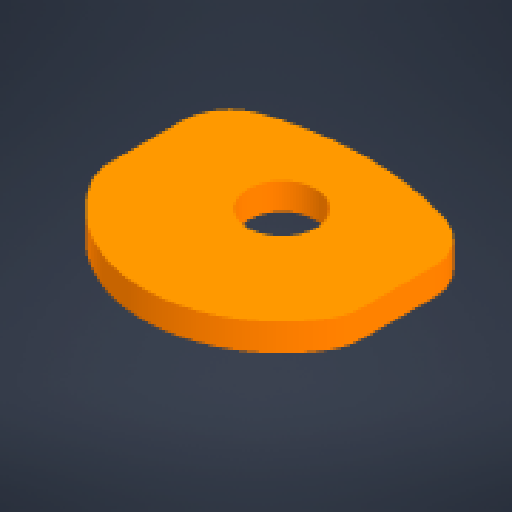
# Autodesk Inventor part: gasket_1
Saved by Autodesk Inventor 2024 (Build 280153000, 153)
## iProperties
Created: 2023-11-08
Part Number: gasket_1
Material: Типовые
Document SubType Name: Modeling
Designer: user
Density: 1 g/cm^3
Appearance: По умолчанию
Author: user
Autodesk Inventor part; units mm, degrees
ref_plane "YZ Plane" through (0, 0, 0) normal (1, 0, 0) x (0, 1, 0)
ref_plane "XZ Plane" through (0, 0, 0) normal (0, 1, 0) x (-1, 0, 0)
ref_plane "XY Plane" through (0, 0, 0) normal (0, 0, 1) x (1, 0, 0)
sketch "Эскиз1" plane through (0, 0, 0) normal (0, 0, 1) x (1, 0, 0)
  circle A0 centre (-3.5, 33.9378) radius 1.5 projected
  circle A1 centre (7, 40) radius 1.5 projected
  circle A2 centre (-7, 40) radius 1.5 projected
  circle A3 centre (3.5, 33.9378) radius 1.5 projected
  arc A4 (9.6, 47.3855) -> (-9.6, 47.3855) centre (0, 18.963) ccw projected
  line L0 (-13, 42.6484) -> (-13, 35.2228) projected
  arc A5 (-12.2928, 32.6593) -> (12.2928, 32.6593) centre (0, 40) ccw projected
  line L1 (13, 35.2228) -> (13, 42.6484) projected
  circle A6 centre (0, 40) radius 3.1 projected
  arc A7 (12.2928, 32.6593) -> (13, 35.2228) centre (8, 35.2228) ccw projected
  arc A8 (13, 42.6484) -> (9.6, 47.3855) centre (8, 42.6484) ccw projected
  arc A9 (-9.6, 47.3855) -> (-13, 42.6484) centre (-8, 42.6484) ccw projected
  arc A10 (-13, 35.2228) -> (-12.2928, 32.6593) centre (-8, 35.2228) ccw projected
  point P0 (0, 0)
extrude "Выдавливание1" add sketch "Эскиз1" against normal blind 3 contours A0 | A1 | A2 | A3
sketch "Эскиз2" plane through (7, 40, 0) normal (0, 0, 1) x (1, 0, 0)
  line L0 (6, -4.7772) -> (6, 2.6484) projected
  arc A0 (-19.2928, -7.3407) -> (5.2928, -7.3407) centre (-7, 0) ccw projected
  line L1 (-20, 2.6484) -> (-20, -4.7772) projected
  arc A1 (2.6, 7.3855) -> (-16.6, 7.3855) centre (-7, -21.037) ccw projected
  circle A2 centre (-7, 0) radius 3.1 construction
  circle A3 centre (-7, 0) radius 3.5
  arc A4 (-16.6, 7.3855) -> (-20, 2.6484) centre (-15, 2.6484) ccw projected
  arc A5 (6, 2.6484) -> (2.6, 7.3855) centre (1, 2.6484) ccw projected
  arc A6 (5.2928, -7.3407) -> (6, -4.7772) centre (1, -4.7772) ccw projected
  arc A7 (-20, -4.7772) -> (-19.2928, -7.3407) centre (-15, -4.7772) ccw projected
  point P0 (-7, -40)
  dimension "d2" = 7
  constraints: 1 centre point, 1 coincident
  measures "d2" diameter of A3
extrude "Выдавливание2" add sketch "Эскиз2" along normal blind 2.8
